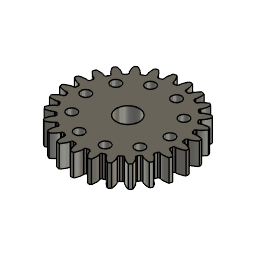
Main gear (Autodesk Fusion 360 design; units mm, degrees)
part number: 2026-05-08-17-31-43-682
Autodesk Fusion 360 part; units mm, degrees
(part 1 of 7)
sketch "Base Circle" plane through (0, 0, 0) normal (0, 0, 1) x (1, 0, 0)
  circle A0 centre (0, 0) radius 11.343
  circle A1 centre (0, 0) radius 2.6
extrude "Extrude6" add sketch "Base Circle" along normal blind 5
sketch "Gear Tooth" plane through (0, 0, 0) normal (0, 0, 1) x (1, 0, 0)
  spline S0 degree 5 poles (11.7116, -0.9005) (11.7167, -0.9009) (11.7269, -0.9015) (11.7422, -0.9021) (11.7626, -0.9022) (11.7882, -0.9014) (11.8137, -0.8998) (11.8394, -0.8977) (11.865, -0.8955) (11.8906, -0.893) (11.9163, -0.8904) (11.9419, -0.8876) (11.9676, -0.8845) (11.9933, -0.8811) (12.0189, -0.8773) (12.0446, -0.8732) (12.0703, -0.8688) (12.096, -0.8641) (12.1216, -0.8593) (12.1473, -0.8543) (12.173, -0.8491) (12.1987, -0.8437) (12.2244, -0.838) (12.25, -0.8322) (12.2757, -0.8262) (12.3014, -0.8199) (12.3271, -0.8135) (12.3527, -0.8068) (12.3784, -0.8) (12.404, -0.793) (12.4297, -0.7859) (12.4553, -0.7785) (12.4809, -0.771) (12.5066, -0.7633) (12.5322, -0.7555) (12.5578, -0.7475) (12.5834, -0.7393) (12.609, -0.7309) (12.6345, -0.7224) (12.6601, -0.7137) (12.6857, -0.7049) (12.7112, -0.6959) (12.7367, -0.6868) (12.7623, -0.6775) (12.7878, -0.668) (12.8133, -0.6584) (12.8387, -0.6487) (12.8642, -0.6388) (12.8897, -0.6287) (12.9151, -0.6185) (12.9405, -0.6082) (12.9659, -0.5977) (12.9913, -0.5871) (13.0167, -0.5764) (13.0421, -0.5655) (13.0674, -0.5544) (13.0928, -0.5433) (13.1181, -0.532) (13.1434, -0.5205) (13.1687, -0.5089) (13.1939, -0.4972) (13.2192, -0.4854) (13.2444, -0.4734) (13.2696, -0.4613) (13.2948, -0.449) (13.32, -0.4366) (13.3451, -0.4241) (13.3702, -0.4115) (13.3953, -0.3987) (13.4204, -0.3858) (13.4455, -0.3728) (13.4655, -0.3623) (13.4805, -0.3544) (13.4906, -0.349) (13.4956, -0.3464) knots 0 0 0 0 0 0 0.01428571 0.02857143 0.04285714 0.05714286 0.07142857 0.08571429 0.1 0.11428571 0.12857143 0.14285714 0.15714286 0.17142857 0.18571429 0.2 0.21428571 0.22857143 0.24285714 0.25714286 0.27142857 0.28571429 0.3 0.31428571 0.32857143 0.34285714 0.35714286 0.37142857 0.38571429 0.4 0.41428571 0.42857143 0.44285714 0.45714286 0.47142857 0.48571429 0.5 0.51428571 0.52857143 0.54285714 0.55714286 0.57142857 0.58571429 0.6 0.61428571 0.62857143 0.64285714 0.65714286 0.67142857 0.68571429 0.7 0.71428571 0.72857143 0.74285714 0.75714286 0.77142857 0.78571429 0.8 0.81428571 0.82857143 0.84285714 0.85714286 0.87142857 0.88571429 0.9 0.91428571 0.92857143 0.94285714 0.95714286 0.97142857 0.98571429 1 1 1 1 1 1
  spline S1 degree 5 poles (11.7116, 0.9005) (11.7167, 0.9009) (11.7269, 0.9015) (11.7422, 0.9021) (11.7626, 0.9022) (11.7882, 0.9014) (11.8137, 0.8998) (11.8394, 0.8977) (11.865, 0.8955) (11.8906, 0.893) (11.9163, 0.8904) (11.9419, 0.8876) (11.9676, 0.8845) (11.9933, 0.8811) (12.0189, 0.8773) (12.0446, 0.8732) (12.0703, 0.8688) (12.096, 0.8641) (12.1216, 0.8593) (12.1473, 0.8543) (12.173, 0.8491) (12.1987, 0.8437) (12.2244, 0.838) (12.25, 0.8322) (12.2757, 0.8262) (12.3014, 0.8199) (12.3271, 0.8135) (12.3527, 0.8068) (12.3784, 0.8) (12.404, 0.793) (12.4297, 0.7859) (12.4553, 0.7785) (12.4809, 0.771) (12.5066, 0.7633) (12.5322, 0.7555) (12.5578, 0.7475) (12.5834, 0.7393) (12.609, 0.7309) (12.6345, 0.7224) (12.6601, 0.7137) (12.6857, 0.7049) (12.7112, 0.6959) (12.7367, 0.6868) (12.7623, 0.6775) (12.7878, 0.668) (12.8133, 0.6584) (12.8387, 0.6487) (12.8642, 0.6388) (12.8897, 0.6287) (12.9151, 0.6185) (12.9405, 0.6082) (12.9659, 0.5977) (12.9913, 0.5871) (13.0167, 0.5764) (13.0421, 0.5655) (13.0674, 0.5544) (13.0928, 0.5433) (13.1181, 0.532) (13.1434, 0.5205) (13.1687, 0.5089) (13.1939, 0.4972) (13.2192, 0.4854) (13.2444, 0.4734) (13.2696, 0.4613) (13.2948, 0.449) (13.32, 0.4366) (13.3451, 0.4241) (13.3702, 0.4115) (13.3953, 0.3987) (13.4204, 0.3858) (13.4455, 0.3728) (13.4655, 0.3623) (13.4805, 0.3544) (13.4906, 0.349) (13.4956, 0.3464) knots 0 0 0 0 0 0 0.01428571 0.02857143 0.04285714 0.05714286 0.07142857 0.08571429 0.1 0.11428571 0.12857143 0.14285714 0.15714286 0.17142857 0.18571429 0.2 0.21428571 0.22857143 0.24285714 0.25714286 0.27142857 0.28571429 0.3 0.31428571 0.32857143 0.34285714 0.35714286 0.37142857 0.38571429 0.4 0.41428571 0.42857143 0.44285714 0.45714286 0.47142857 0.48571429 0.5 0.51428571 0.52857143 0.54285714 0.55714286 0.57142857 0.58571429 0.6 0.61428571 0.62857143 0.64285714 0.65714286 0.67142857 0.68571429 0.7 0.71428571 0.72857143 0.74285714 0.75714286 0.77142857 0.78571429 0.8 0.81428571 0.82857143 0.84285714 0.85714286 0.87142857 0.88571429 0.9 0.91428571 0.92857143 0.94285714 0.95714286 0.97142857 0.98571429 1 1 1 1 1 1
  arc A0 (13.4956, -0.3464) -> (13.4956, 0.3464) centre (0, 0) ccw
  line L0 (11.2996, -0.8688) -> (11.7116, -0.9005)
  line L1 (11.2996, 0.8688) -> (11.7116, 0.9005)
  line L2 (11.2996, -0.8688) -> (11.2996, 0.8688)
  point P0 (11.8374, -0.8978)
  point P1 (11.964, -0.8849)
  point P2 (12.0911, -0.865)
  point P3 (12.2185, -0.8393)
  point P4 (12.3461, -0.8085)
  point P5 (12.4739, -0.7731)
  point P6 (12.6018, -0.7332)
  point P7 (12.7297, -0.6892)
  point P8 (12.8576, -0.6413)
  point P9 (12.9855, -0.5895)
  point P10 (13.1133, -0.5341)
  point P11 (13.2409, -0.475)
  point P12 (13.3684, -0.4124)
  point P13 (11.8374, 0.8978)
  point P14 (11.964, 0.8849)
  point P15 (12.0911, 0.865)
  point P16 (12.2185, 0.8393)
  point P17 (12.3461, 0.8085)
  point P18 (12.4739, 0.7731)
  point P19 (12.6018, 0.7332)
  point P20 (12.7297, 0.6892)
  point P21 (12.8576, 0.6413)
  point P22 (12.9855, 0.5895)
  point P23 (13.1133, 0.5341)
  point P24 (13.2409, 0.475)
  point P25 (13.3684, 0.4124)
extrude "Extrude7" add sketch "Gear Tooth" along normal blind 5
fillet "Fillet3" radius 0.3 2 edges at (11.3096, -0.8696, 2.5) (11.3096, 0.8696, 2.5)
pattern_circular "C-Pattern3" count 25 over 360 about axis through (0, 0, 0) along (0, 0, 1) of "Extrude7", "Fillet3"
sketch "Diametrial Pitch Circle" plane through (0, 0, 0) normal (0, 0, 1) x (1, 0, 0)
  circle A0 centre (0, 0) radius 12.5 construction
sketch "gauri flaps" plane through (0, 0, 5) normal (0, 0, 1) x (-1, 0, 0)
  arc A0 (-11.2176, 1.6819) -> (-11.2835, 1.1607) centre (0, 0) ccw
  arc A1 (-11.6049, 0.8923) -> (-11.2835, 1.1607) centre (-11.5819, 1.1914) ccw
  line L0 (-11.6049, 0.8923) -> (-11.7116, 0.9005)
  spline S0 degree 5 poles (-11.7116, 0.9005) (-11.7167, 0.9009) (-11.7269, 0.9015) (-11.7422, 0.9021) (-11.7626, 0.9022) (-11.7882, 0.9014) (-11.8137, 0.8998) (-11.8394, 0.8977) (-11.865, 0.8955) (-11.8906, 0.893) (-11.9163, 0.8904) (-11.9419, 0.8876) (-11.9676, 0.8845) (-11.9933, 0.8811) (-12.0189, 0.8773) (-12.0446, 0.8732) (-12.0703, 0.8688) (-12.096, 0.8641) (-12.1216, 0.8593) (-12.1473, 0.8543) (-12.173, 0.8491) (-12.1987, 0.8437) (-12.2244, 0.838) (-12.25, 0.8322) (-12.2757, 0.8262) (-12.3014, 0.8199) (-12.3271, 0.8135) (-12.3527, 0.8068) (-12.3784, 0.8) (-12.404, 0.793) (-12.4297, 0.7859) (-12.4553, 0.7785) (-12.4809, 0.771) (-12.5066, 0.7633) (-12.5322, 0.7555) (-12.5578, 0.7475) (-12.5834, 0.7393) (-12.609, 0.7309) (-12.6345, 0.7224) (-12.6601, 0.7137) (-12.6857, 0.7049) (-12.7112, 0.6959) (-12.7367, 0.6868) (-12.7623, 0.6775) (-12.7878, 0.668) (-12.8133, 0.6584) (-12.8387, 0.6487) (-12.8642, 0.6388) (-12.8897, 0.6287) (-12.9151, 0.6185) (-12.9405, 0.6082) (-12.9659, 0.5977) (-12.9913, 0.5871) (-13.0167, 0.5764) (-13.0421, 0.5655) (-13.0674, 0.5544) (-13.0928, 0.5433) (-13.1181, 0.532) (-13.1434, 0.5205) (-13.1687, 0.5089) (-13.1939, 0.4972) (-13.2192, 0.4854) (-13.2444, 0.4734) (-13.2696, 0.4613) (-13.2948, 0.449) (-13.32, 0.4366) (-13.3451, 0.4241) (-13.3702, 0.4115) (-13.3953, 0.3987) (-13.4204, 0.3858) (-13.4455, 0.3728) (-13.4655, 0.3623) (-13.4805, 0.3544) (-13.4906, 0.349) (-13.4956, 0.3464) knots 0 0 0 0 0 0 0.01428571 0.02857143 0.04285714 0.05714286 0.07142857 0.08571429 0.1 0.11428571 0.12857143 0.14285714 0.15714286 0.17142857 0.18571429 0.2 0.21428571 0.22857143 0.24285714 0.25714286 0.27142857 0.28571429 0.3 0.31428571 0.32857143 0.34285714 0.35714286 0.37142857 0.38571429 0.4 0.41428571 0.42857143 0.44285714 0.45714286 0.47142857 0.48571429 0.5 0.51428571 0.52857143 0.54285714 0.55714286 0.57142857 0.58571429 0.6 0.61428571 0.62857143 0.64285714 0.65714286 0.67142857 0.68571429 0.7 0.71428571 0.72857143 0.74285714 0.75714286 0.77142857 0.78571429 0.8 0.81428571 0.82857143 0.84285714 0.85714286 0.87142857 0.88571429 0.9 0.91428571 0.92857143 0.94285714 0.95714286 0.97142857 0.98571429 1 1 1 1 1 1
  arc A2 (-13.4956, 0.3464) -> (-13.4956, -0.3464) centre (0, 0) ccw
  spline S1 degree 5 poles (-13.4956, -0.3464) (-13.4906, -0.349) (-13.4805, -0.3544) (-13.4655, -0.3623) (-13.4455, -0.3728) (-13.4204, -0.3858) (-13.3953, -0.3987) (-13.3702, -0.4115) (-13.3451, -0.4241) (-13.32, -0.4366) (-13.2948, -0.449) (-13.2696, -0.4613) (-13.2444, -0.4734) (-13.2192, -0.4854) (-13.1939, -0.4972) (-13.1687, -0.5089) (-13.1434, -0.5205) (-13.1181, -0.532) (-13.0928, -0.5433) (-13.0674, -0.5544) (-13.0421, -0.5655) (-13.0167, -0.5764) (-12.9913, -0.5871) (-12.9659, -0.5977) (-12.9405, -0.6082) (-12.9151, -0.6185) (-12.8897, -0.6287) (-12.8642, -0.6388) (-12.8387, -0.6487) (-12.8133, -0.6584) (-12.7878, -0.668) (-12.7623, -0.6775) (-12.7367, -0.6868) (-12.7112, -0.6959) (-12.6857, -0.7049) (-12.6601, -0.7137) (-12.6345, -0.7224) (-12.609, -0.7309) (-12.5834, -0.7393) (-12.5578, -0.7475) (-12.5322, -0.7555) (-12.5066, -0.7633) (-12.4809, -0.771) (-12.4553, -0.7785) (-12.4297, -0.7859) (-12.404, -0.793) (-12.3784, -0.8) (-12.3527, -0.8068) (-12.3271, -0.8135) (-12.3014, -0.8199) (-12.2757, -0.8262) (-12.25, -0.8322) (-12.2244, -0.838) (-12.1987, -0.8437) (-12.173, -0.8491) (-12.1473, -0.8543) (-12.1216, -0.8593) (-12.096, -0.8641) (-12.0703, -0.8688) (-12.0446, -0.8732) (-12.0189, -0.8773) (-11.9933, -0.8811) (-11.9676, -0.8845) (-11.9419, -0.8876) (-11.9163, -0.8904) (-11.8906, -0.893) (-11.865, -0.8955) (-11.8394, -0.8977) (-11.8137, -0.8998) (-11.7882, -0.9014) (-11.7626, -0.9022) (-11.7422, -0.9021) (-11.7269, -0.9015) (-11.7167, -0.9009) (-11.7116, -0.9005) knots -1 -1 -1 -1 -1 -1 -0.98571429 -0.97142857 -0.95714286 -0.94285714 -0.92857143 -0.91428571 -0.9 -0.88571429 -0.87142857 -0.85714286 -0.84285714 -0.82857143 -0.81428571 -0.8 -0.78571429 -0.77142857 -0.75714286 -0.74285714 -0.72857143 -0.71428571 -0.7 -0.68571429 -0.67142857 -0.65714286 -0.64285714 -0.62857143 -0.61428571 -0.6 -0.58571429 -0.57142857 -0.55714286 -0.54285714 -0.52857143 -0.51428571 -0.5 -0.48571429 -0.47142857 -0.45714286 -0.44285714 -0.42857143 -0.41428571 -0.4 -0.38571429 -0.37142857 -0.35714286 -0.34285714 -0.32857143 -0.31428571 -0.3 -0.28571429 -0.27142857 -0.25714286 -0.24285714 -0.22857143 -0.21428571 -0.2 -0.18571429 -0.17142857 -0.15714286 -0.14285714 -0.12857143 -0.11428571 -0.1 -0.08571429 -0.07142857 -0.05714286 -0.04285714 -0.02857143 -0.01428571 0 0 0 0 0 0
  line L1 (-11.7116, -0.9005) -> (-11.6049, -0.8923)
  arc A3 (-11.2835, -1.1607) -> (-11.6049, -0.8923) centre (-11.5819, -1.1914) ccw
  arc A4 (-11.2835, -1.1607) -> (-11.2176, -1.6819) centre (0, 0) ccw
  arc A5 (-11.4622, -2.0218) -> (-11.2176, -1.6819) centre (-11.5143, -1.7263) ccw
  line L2 (-11.4622, -2.0218) -> (-11.5676, -2.0404)
  spline S2 degree 5 poles (-11.5676, -2.0404) (-11.5726, -2.0413) (-11.5827, -2.0432) (-11.5976, -2.0464) (-11.6174, -2.0514) (-11.642, -2.0586) (-11.6664, -2.0665) (-11.6907, -2.0748) (-11.7149, -2.0834) (-11.7391, -2.0921) (-11.7633, -2.101) (-11.7875, -2.1101) (-11.8116, -2.1195) (-11.8356, -2.1292) (-11.8595, -2.1393) (-11.8833, -2.1496) (-11.9071, -2.1603) (-11.9308, -2.1712) (-11.9545, -2.1822) (-11.9781, -2.1935) (-12.0017, -2.2049) (-12.0253, -2.2165) (-12.0487, -2.2284) (-12.0722, -2.2404) (-12.0955, -2.2526) (-12.1188, -2.2651) (-12.1421, -2.2777) (-12.1653, -2.2905) (-12.1884, -2.3035) (-12.2115, -2.3166) (-12.2346, -2.33) (-12.2576, -2.3434) (-12.2806, -2.3571) (-12.3035, -2.3709) (-12.3263, -2.3849) (-12.3491, -2.399) (-12.3719, -2.4133) (-12.3946, -2.4278) (-12.4172, -2.4424) (-12.4399, -2.4571) (-12.4624, -2.4721) (-12.4849, -2.4871) (-12.5074, -2.5023) (-12.5298, -2.5177) (-12.5521, -2.5332) (-12.5744, -2.5488) (-12.5967, -2.5646) (-12.6189, -2.5805) (-12.6411, -2.5965) (-12.6632, -2.6127) (-12.6852, -2.6291) (-12.7072, -2.6455) (-12.7292, -2.6621) (-12.7511, -2.6789) (-12.773, -2.6957) (-12.7948, -2.7127) (-12.8165, -2.7298) (-12.8382, -2.7471) (-12.8599, -2.7645) (-12.8815, -2.782) (-12.9031, -2.7996) (-12.9246, -2.8174) (-12.946, -2.8352) (-12.9674, -2.8532) (-12.9888, -2.8714) (-13.0101, -2.8896) (-13.0313, -2.908) (-13.0525, -2.9265) (-13.0737, -2.9451) (-13.0948, -2.9638) (-13.1158, -2.9827) (-13.1326, -2.9978) (-13.1452, -3.0092) (-13.1535, -3.0169) (-13.1577, -3.0207) knots 0 0 0 0 0 0 0.01428571 0.02857143 0.04285714 0.05714286 0.07142857 0.08571429 0.1 0.11428571 0.12857143 0.14285714 0.15714286 0.17142857 0.18571429 0.2 0.21428571 0.22857143 0.24285714 0.25714286 0.27142857 0.28571429 0.3 0.31428571 0.32857143 0.34285714 0.35714286 0.37142857 0.38571429 0.4 0.41428571 0.42857143 0.44285714 0.45714286 0.47142857 0.48571429 0.5 0.51428571 0.52857143 0.54285714 0.55714286 0.57142857 0.58571429 0.6 0.61428571 0.62857143 0.64285714 0.65714286 0.67142857 0.68571429 0.7 0.71428571 0.72857143 0.74285714 0.75714286 0.77142857 0.78571429 0.8 0.81428571 0.82857143 0.84285714 0.85714286 0.87142857 0.88571429 0.9 0.91428571 0.92857143 0.94285714 0.95714286 0.97142857 0.98571429 1 1 1 1 1 1
  arc A6 (-13.1577, -3.0207) -> (-12.9854, -3.6917) centre (0, 0) ccw
  spline S3 degree 5 poles (-12.9854, -3.6917) (-12.9799, -3.693) (-12.9689, -3.6957) (-12.9524, -3.6997) (-12.9304, -3.7049) (-12.9028, -3.7112) (-12.8753, -3.7175) (-12.8478, -3.7236) (-12.8204, -3.7296) (-12.7929, -3.7355) (-12.7654, -3.7412) (-12.738, -3.7468) (-12.7106, -3.7522) (-12.6832, -3.7576) (-12.6558, -3.7628) (-12.6284, -3.7678) (-12.601, -3.7728) (-12.5737, -3.7776) (-12.5463, -3.7822) (-12.519, -3.7868) (-12.4917, -3.7911) (-12.4644, -3.7954) (-12.4372, -3.7995) (-12.4099, -3.8035) (-12.3827, -3.8073) (-12.3555, -3.811) (-12.3283, -3.8145) (-12.3012, -3.8179) (-12.2741, -3.8212) (-12.247, -3.8243) (-12.2199, -3.8272) (-12.1928, -3.83) (-12.1658, -3.8327) (-12.1388, -3.8352) (-12.1118, -3.8375) (-12.0849, -3.8397) (-12.0579, -3.8418) (-12.0311, -3.8437) (-12.0042, -3.8454) (-11.9774, -3.847) (-11.9506, -3.8484) (-11.9238, -3.8496) (-11.8971, -3.8507) (-11.8704, -3.8516) (-11.8437, -3.8523) (-11.8171, -3.8529) (-11.7905, -3.8533) (-11.764, -3.8535) (-11.7375, -3.8535) (-11.711, -3.8534) (-11.6846, -3.8531) (-11.6582, -3.8525) (-11.6319, -3.8518) (-11.6056, -3.8508) (-11.5794, -3.8497) (-11.5532, -3.8484) (-11.5271, -3.8468) (-11.501, -3.8451) (-11.475, -3.8432) (-11.4491, -3.8411) (-11.4232, -3.8387) (-11.3974, -3.836) (-11.3716, -3.8329) (-11.346, -3.8296) (-11.3205, -3.8259) (-11.295, -3.8221) (-11.2695, -3.818) (-11.2441, -3.8139) (-11.2188, -3.8095) (-11.1937, -3.8046) (-11.1687, -3.7991) (-11.1489, -3.794) (-11.1343, -3.7896) (-11.1245, -3.7864) (-11.1197, -3.7847) knots -1 -1 -1 -1 -1 -1 -0.98571429 -0.97142857 -0.95714286 -0.94285714 -0.92857143 -0.91428571 -0.9 -0.88571429 -0.87142857 -0.85714286 -0.84285714 -0.82857143 -0.81428571 -0.8 -0.78571429 -0.77142857 -0.75714286 -0.74285714 -0.72857143 -0.71428571 -0.7 -0.68571429 -0.67142857 -0.65714286 -0.64285714 -0.62857143 -0.61428571 -0.6 -0.58571429 -0.57142857 -0.55714286 -0.54285714 -0.52857143 -0.51428571 -0.5 -0.48571429 -0.47142857 -0.45714286 -0.44285714 -0.42857143 -0.41428571 -0.4 -0.38571429 -0.37142857 -0.35714286 -0.34285714 -0.32857143 -0.31428571 -0.3 -0.28571429 -0.27142857 -0.25714286 -0.24285714 -0.22857143 -0.21428571 -0.2 -0.18571429 -0.17142857 -0.15714286 -0.14285714 -0.12857143 -0.11428571 -0.1 -0.08571429 -0.07142857 -0.05714286 -0.04285714 -0.02857143 -0.01428571 0 0 0 0 0 0
  line L3 (-11.1197, -3.7847) -> (-11.0184, -3.7503)
  arc A7 (-10.6403, -3.9303) -> (-11.0184, -3.7503) centre (-10.9217, -4.0343) ccw
  arc A8 (-10.6403, -3.9303) -> (-10.4469, -4.4187) centre (0, 0) ccw
  arc A9 (-10.5993, -4.8088) -> (-10.4469, -4.4187) centre (-10.7232, -4.5356) ccw
  line L4 (-10.5993, -4.8088) -> (-10.6968, -4.853)
  spline S4 degree 5 poles (-10.6968, -4.853) (-10.7014, -4.8551) (-10.7107, -4.8595) (-10.7244, -4.8663) (-10.7423, -4.8761) (-10.7643, -4.8891) (-10.7859, -4.9028) (-10.8074, -4.917) (-10.8288, -4.9313) (-10.85, -4.9458) (-10.8713, -4.9604) (-10.8924, -4.9752) (-10.9134, -4.9903) (-10.9342, -5.0057) (-10.9549, -5.0214) (-10.9754, -5.0374) (-10.9958, -5.0536) (-11.0161, -5.07) (-11.0362, -5.0866) (-11.0563, -5.1034) (-11.0763, -5.1203) (-11.0962, -5.1375) (-11.116, -5.1547) (-11.1357, -5.1722) (-11.1553, -5.1899) (-11.1748, -5.2077) (-11.1942, -5.2258) (-11.2135, -5.2439) (-11.2327, -5.2623) (-11.2518, -5.2807) (-11.2708, -5.2994) (-11.2897, -5.3182) (-11.3086, -5.3371) (-11.3273, -5.3562) (-11.346, -5.3754) (-11.3646, -5.3948) (-11.383, -5.4143) (-11.4014, -5.4339) (-11.4197, -5.4537) (-11.438, -5.4736) (-11.4561, -5.4937) (-11.4742, -5.5138) (-11.4921, -5.5342) (-11.51, -5.5546) (-11.5278, -5.5752) (-11.5455, -5.5959) (-11.5632, -5.6167) (-11.5807, -5.6376) (-11.5982, -5.6587) (-11.6156, -5.6799) (-11.6329, -5.7012) (-11.6501, -5.7226) (-11.6672, -5.7441) (-11.6843, -5.7658) (-11.7013, -5.7875) (-11.7182, -5.8094) (-11.735, -5.8314) (-11.7517, -5.8535) (-11.7684, -5.8757) (-11.785, -5.8981) (-11.8015, -5.9205) (-11.8179, -5.9431) (-11.8342, -5.9657) (-11.8505, -5.9885) (-11.8666, -6.0113) (-11.8827, -6.0343) (-11.8987, -6.0574) (-11.9147, -6.0806) (-11.9305, -6.1038) (-11.9463, -6.1272) (-11.962, -6.1507) (-11.9745, -6.1696) (-11.9838, -6.1838) (-11.99, -6.1933) (-11.9931, -6.198) knots 0 0 0 0 0 0 0.01428571 0.02857143 0.04285714 0.05714286 0.07142857 0.08571429 0.1 0.11428571 0.12857143 0.14285714 0.15714286 0.17142857 0.18571429 0.2 0.21428571 0.22857143 0.24285714 0.25714286 0.27142857 0.28571429 0.3 0.31428571 0.32857143 0.34285714 0.35714286 0.37142857 0.38571429 0.4 0.41428571 0.42857143 0.44285714 0.45714286 0.47142857 0.48571429 0.5 0.51428571 0.52857143 0.54285714 0.55714286 0.57142857 0.58571429 0.6 0.61428571 0.62857143 0.64285714 0.65714286 0.67142857 0.68571429 0.7 0.71428571 0.72857143 0.74285714 0.75714286 0.77142857 0.78571429 0.8 0.81428571 0.82857143 0.84285714 0.85714286 0.87142857 0.88571429 0.9 0.91428571 0.92857143 0.94285714 0.95714286 0.97142857 0.98571429 1 1 1 1 1 1
  arc A10 (-11.9931, -6.198) -> (-11.6594, -6.8051) centre (0, 0) ccw
  spline S5 degree 5 poles (-11.6594, -6.8051) (-11.6537, -6.805) (-11.6424, -6.8048) (-11.6254, -6.8046) (-11.6028, -6.8041) (-11.5745, -6.8035) (-11.5463, -6.8027) (-11.5182, -6.8018) (-11.4901, -6.8007) (-11.462, -6.7996) (-11.434, -6.7983) (-11.406, -6.7969) (-11.3781, -6.7954) (-11.3502, -6.7937) (-11.3224, -6.7919) (-11.2946, -6.79) (-11.2669, -6.788) (-11.2392, -6.7858) (-11.2116, -6.7836) (-11.184, -6.7811) (-11.1564, -6.7786) (-11.129, -6.7759) (-11.1015, -6.7731) (-11.0742, -6.7702) (-11.0469, -6.7671) (-11.0196, -6.7639) (-10.9924, -6.7606) (-10.9653, -6.7571) (-10.9382, -6.7535) (-10.9111, -6.7498) (-10.8842, -6.7459) (-10.8573, -6.7419) (-10.8304, -6.7378) (-10.8037, -6.7335) (-10.7769, -6.7291) (-10.7503, -6.7245) (-10.7237, -6.7198) (-10.6972, -6.7149) (-10.6707, -6.7099) (-10.6444, -6.7048) (-10.6181, -6.6995) (-10.5918, -6.694) (-10.5657, -6.6884) (-10.5396, -6.6826) (-10.5136, -6.6767) (-10.4877, -6.6706) (-10.4618, -6.6644) (-10.4361, -6.658) (-10.4104, -6.6515) (-10.3848, -6.6447) (-10.3593, -6.6379) (-10.3339, -6.6308) (-10.3086, -6.6235) (-10.2834, -6.6161) (-10.2582, -6.6084) (-10.2332, -6.6006) (-10.2083, -6.5927) (-10.1835, -6.5845) (-10.1587, -6.5762) (-10.1341, -6.5677) (-10.1096, -6.5589) (-10.0853, -6.5499) (-10.0612, -6.5405) (-10.0372, -6.5309) (-10.0133, -6.521) (-9.9896, -6.5109) (-9.966, -6.5007) (-9.9424, -6.4904) (-9.919, -6.4798) (-9.8958, -6.4689) (-9.873, -6.4573) (-9.8551, -6.4474) (-9.842, -6.4395) (-9.8334, -6.434) (-9.8291, -6.4312) knots -1 -1 -1 -1 -1 -1 -0.98571429 -0.97142857 -0.95714286 -0.94285714 -0.92857143 -0.91428571 -0.9 -0.88571429 -0.87142857 -0.85714286 -0.84285714 -0.82857143 -0.81428571 -0.8 -0.78571429 -0.77142857 -0.75714286 -0.74285714 -0.72857143 -0.71428571 -0.7 -0.68571429 -0.67142857 -0.65714286 -0.64285714 -0.62857143 -0.61428571 -0.6 -0.58571429 -0.57142857 -0.55714286 -0.54285714 -0.52857143 -0.51428571 -0.5 -0.48571429 -0.47142857 -0.45714286 -0.44285714 -0.42857143 -0.41428571 -0.4 -0.38571429 -0.37142857 -0.35714286 -0.34285714 -0.32857143 -0.31428571 -0.3 -0.28571429 -0.27142857 -0.25714286 -0.24285714 -0.22857143 -0.21428571 -0.2 -0.18571429 -0.17142857 -0.15714286 -0.14285714 -0.12857143 -0.11428571 -0.1 -0.08571429 -0.07142857 -0.05714286 -0.04285714 -0.02857143 -0.01428571 0 0 0 0 0 0
  line L5 (-9.8291, -6.4312) -> (-9.7396, -6.3726)
  arc A11 (-9.3286, -6.453) -> (-9.7396, -6.3726) centre (-9.5753, -6.6236) ccw
  arc A12 (-9.3286, -6.453) -> (-9.0198, -6.878) centre (0, 0) ccw
  arc A13 (-9.0704, -7.2937) -> (-9.0198, -6.878) centre (-9.2584, -7.0599) ccw
  line L6 (-9.0704, -7.2937) -> (-9.1538, -7.3607)
  spline S6 degree 5 poles (-9.1538, -7.3607) (-9.1578, -7.3639) (-9.1657, -7.3704) (-9.1772, -7.3805) (-9.1922, -7.3944) (-9.2102, -7.4125) (-9.2278, -7.4312) (-9.2451, -7.4502) (-9.2622, -7.4694) (-9.2792, -7.4887) (-9.2961, -7.5081) (-9.3129, -7.5278) (-9.3295, -7.5476) (-9.3458, -7.5677) (-9.362, -7.588) (-9.3779, -7.6086) (-9.3936, -7.6294) (-9.4091, -7.6503) (-9.4245, -7.6714) (-9.4398, -7.6927) (-9.455, -7.7141) (-9.47, -7.7356) (-9.4849, -7.7572) (-9.4996, -7.7791) (-9.5142, -7.8011) (-9.5286, -7.8232) (-9.5429, -7.8455) (-9.5571, -7.8679) (-9.5711, -7.8904) (-9.585, -7.913) (-9.5988, -7.9358) (-9.6125, -7.9587) (-9.626, -7.9817) (-9.6394, -8.0049) (-9.6527, -8.0281) (-9.6659, -8.0515) (-9.6789, -8.075) (-9.6919, -8.0986) (-9.7047, -8.1223) (-9.7174, -8.1462) (-9.73, -8.1701) (-9.7424, -8.1941) (-9.7548, -8.2183) (-9.767, -8.2425) (-9.7792, -8.2669) (-9.7912, -8.2913) (-9.8031, -8.3159) (-9.8149, -8.3405) (-9.8266, -8.3653) (-9.8381, -8.3901) (-9.8496, -8.415) (-9.8609, -8.4401) (-9.8722, -8.4652) (-9.8833, -8.4904) (-9.8944, -8.5157) (-9.9053, -8.5411) (-9.9161, -8.5666) (-9.9268, -8.5922) (-9.9374, -8.6178) (-9.9479, -8.6436) (-9.9583, -8.6694) (-9.9686, -8.6953) (-9.9788, -8.7213) (-9.9889, -8.7474) (-9.9989, -8.7736) (-10.0087, -8.7998) (-10.0185, -8.8262) (-10.0282, -8.8526) (-10.0377, -8.8791) (-10.0472, -8.9057) (-10.0566, -8.9323) (-10.064, -8.9537) (-10.0695, -8.9698) (-10.0731, -8.9805) (-10.0749, -8.9858) knots 0 0 0 0 0 0 0.01428571 0.02857143 0.04285714 0.05714286 0.07142857 0.08571429 0.1 0.11428571 0.12857143 0.14285714 0.15714286 0.17142857 0.18571429 0.2 0.21428571 0.22857143 0.24285714 0.25714286 0.27142857 0.28571429 0.3 0.31428571 0.32857143 0.34285714 0.35714286 0.37142857 0.38571429 0.4 0.41428571 0.42857143 0.44285714 0.45714286 0.47142857 0.48571429 0.5 0.51428571 0.52857143 0.54285714 0.55714286 0.57142857 0.58571429 0.6 0.61428571 0.62857143 0.64285714 0.65714286 0.67142857 0.68571429 0.7 0.71428571 0.72857143 0.74285714 0.75714286 0.77142857 0.78571429 0.8 0.81428571 0.82857143 0.84285714 0.85714286 0.87142857 0.88571429 0.9 0.91428571 0.92857143 0.94285714 0.95714286 0.97142857 0.98571429 1 1 1 1 1 1
  arc A14 (-10.0749, -8.9858) -> (-9.6007, -9.4908) centre (0, 0) ccw
  spline S7 degree 5 poles (-9.6007, -9.4908) (-9.5953, -9.4894) (-9.5843, -9.4864) (-9.5679, -9.4819) (-9.5461, -9.4758) (-9.5189, -9.4682) (-9.4918, -9.4604) (-9.4648, -9.4525) (-9.4378, -9.4445) (-9.4109, -9.4364) (-9.3841, -9.4282) (-9.3574, -9.4199) (-9.3307, -9.4115) (-9.3041, -9.403) (-9.2776, -9.3943) (-9.2512, -9.3856) (-9.2248, -9.3767) (-9.1985, -9.3677) (-9.1723, -9.3586) (-9.1462, -9.3494) (-9.1202, -9.3401) (-9.0942, -9.3307) (-9.0684, -9.3212) (-9.0426, -9.3115) (-9.0169, -9.3018) (-8.9913, -9.2919) (-8.9658, -9.2819) (-8.9403, -9.2718) (-8.915, -9.2616) (-8.8897, -9.2512) (-8.8646, -9.2408) (-8.8395, -9.2302) (-8.8146, -9.2195) (-8.7897, -9.2087) (-8.7649, -9.1978) (-8.7402, -9.1867) (-8.7157, -9.1755) (-8.6912, -9.1642) (-8.6668, -9.1528) (-8.6426, -9.1413) (-8.6184, -9.1296) (-8.5943, -9.1178) (-8.5704, -9.1058) (-8.5466, -9.0938) (-8.5229, -9.0816) (-8.4993, -9.0692) (-8.4758, -9.0568) (-8.4524, -9.0442) (-8.4292, -9.0314) (-8.4061, -9.0186) (-8.3831, -9.0056) (-8.3602, -8.9924) (-8.3375, -8.9791) (-8.3149, -8.9656) (-8.2925, -8.9519) (-8.2702, -8.9382) (-8.2481, -8.9242) (-8.226, -8.9102) (-8.2042, -8.896) (-8.1824, -8.8816) (-8.1609, -8.867) (-8.1396, -8.8522) (-8.1185, -8.8372) (-8.0977, -8.8219) (-8.077, -8.8063) (-8.0566, -8.7907) (-8.0362, -8.7749) (-8.016, -8.759) (-7.9959, -8.743) (-7.9762, -8.7266) (-7.957, -8.7098) (-7.9421, -8.6957) (-7.9314, -8.6848) (-7.9244, -8.6773) (-7.921, -8.6736) knots -1 -1 -1 -1 -1 -1 -0.98571429 -0.97142857 -0.95714286 -0.94285714 -0.92857143 -0.91428571 -0.9 -0.88571429 -0.87142857 -0.85714286 -0.84285714 -0.82857143 -0.81428571 -0.8 -0.78571429 -0.77142857 -0.75714286 -0.74285714 -0.72857143 -0.71428571 -0.7 -0.68571429 -0.67142857 -0.65714286 -0.64285714 -0.62857143 -0.61428571 -0.6 -0.58571429 -0.57142857 -0.55714286 -0.54285714 -0.52857143 -0.51428571 -0.5 -0.48571429 -0.47142857 -0.45714286 -0.44285714 -0.42857143 -0.41428571 -0.4 -0.38571429 -0.37142857 -0.35714286 -0.34285714 -0.32857143 -0.31428571 -0.3 -0.28571429 -0.27142857 -0.25714286 -0.24285714 -0.22857143 -0.21428571 -0.2 -0.18571429 -0.17142857 -0.15714286 -0.14285714 -0.12857143 -0.11428571 -0.1 -0.08571429 -0.07142857 -0.05714286 -0.04285714 -0.02857143 -0.01428571 0 0 0 0 0 0
  line L7 (-7.921, -8.6736) -> (-7.8488, -8.5945)
  arc A15 (-7.4307, -8.5702) -> (-7.8488, -8.5945) centre (-7.6273, -8.7968) ccw
  arc A16 (-7.4307, -8.5702) -> (-7.026, -8.905) centre (0, 0) ccw
  arc A17 (-6.9716, -9.3202) -> (-7.026, -8.905) centre (-7.2118, -9.1405) ccw
  line L8 (-6.9716, -9.3202) -> (-7.0357, -9.4059)
  spline S8 degree 5 poles (-7.0357, -9.4059) (-7.0387, -9.41) (-7.0448, -9.4183) (-7.0535, -9.4309) (-7.0645, -9.4481) (-7.0775, -9.4701) (-7.0898, -9.4926) (-7.1018, -9.5153) (-7.1136, -9.5381) (-7.1253, -9.5611) (-7.1369, -9.5841) (-7.1482, -9.6073) (-7.1594, -9.6306) (-7.1702, -9.6541) (-7.1808, -9.6778) (-7.191, -9.7017) (-7.2011, -9.7258) (-7.2109, -9.7499) (-7.2206, -9.7742) (-7.2302, -9.7986) (-7.2395, -9.8231) (-7.2487, -9.8476) (-7.2577, -9.8723) (-7.2666, -9.8971) (-7.2752, -9.9221) (-7.2837, -9.9471) (-7.292, -9.9722) (-7.3002, -9.9974) (-7.3081, -10.0227) (-7.316, -10.0481) (-7.3237, -10.0736) (-7.3312, -10.0992) (-7.3386, -10.1249) (-7.3459, -10.1506) (-7.3529, -10.1765) (-7.3599, -10.2024) (-7.3667, -10.2284) (-7.3733, -10.2545) (-7.3799, -10.2806) (-7.3862, -10.3068) (-7.3925, -10.3332) (-7.3986, -10.3595) (-7.4045, -10.386) (-7.4104, -10.4125) (-7.416, -10.4391) (-7.4216, -10.4658) (-7.427, -10.4925) (-7.4323, -10.5193) (-7.4375, -10.5462) (-7.4425, -10.5731) (-7.4474, -10.6002) (-7.4522, -10.6272) (-7.4568, -10.6544) (-7.4614, -10.6815) (-7.4657, -10.7088) (-7.47, -10.7361) (-7.4741, -10.7635) (-7.4782, -10.7909) (-7.4821, -10.8184) (-7.4858, -10.846) (-7.4895, -10.8736) (-7.493, -10.9012) (-7.4964, -10.929) (-7.4997, -10.9567) (-7.5028, -10.9846) (-7.5059, -11.0125) (-7.5088, -11.0404) (-7.5116, -11.0684) (-7.5142, -11.0964) (-7.5168, -11.1245) (-7.5192, -11.1526) (-7.5211, -11.1752) (-7.5224, -11.1921) (-7.5233, -11.2034) (-7.5237, -11.2091) knots 0 0 0 0 0 0 0.01428571 0.02857143 0.04285714 0.05714286 0.07142857 0.08571429 0.1 0.11428571 0.12857143 0.14285714 0.15714286 0.17142857 0.18571429 0.2 0.21428571 0.22857143 0.24285714 0.25714286 0.27142857 0.28571429 0.3 0.31428571 0.32857143 0.34285714 0.35714286 0.37142857 0.38571429 0.4 0.41428571 0.42857143 0.44285714 0.45714286 0.47142857 0.48571429 0.5 0.51428571 0.52857143 0.54285714 0.55714286 0.57142857 0.58571429 0.6 0.61428571 0.62857143 0.64285714 0.65714286 0.67142857 0.68571429 0.7 0.71428571 0.72857143 0.74285714 0.75714286 0.77142857 0.78571429 0.8 0.81428571 0.82857143 0.84285714 0.85714286 0.87142857 0.88571429 0.9 0.91428571 0.92857143 0.94285714 0.95714286 0.97142857 0.98571429 1 1 1 1 1 1
  arc A18 (-7.5237, -11.2091) -> (-6.9388, -11.5803) centre (0, 0) ccw
  spline S9 degree 5 poles (-6.9388, -11.5803) (-6.9339, -11.5775) (-6.924, -11.5719) (-6.9093, -11.5635) (-6.8897, -11.5522) (-6.8653, -11.538) (-6.8409, -11.5237) (-6.8167, -11.5094) (-6.7926, -11.4949) (-6.7685, -11.4804) (-6.7446, -11.4658) (-6.7208, -11.451) (-6.697, -11.4363) (-6.6734, -11.4214) (-6.6499, -11.4064) (-6.6264, -11.3914) (-6.6031, -11.3762) (-6.5799, -11.361) (-6.5568, -11.3457) (-6.5338, -11.3303) (-6.5109, -11.3148) (-6.4881, -11.2992) (-6.4654, -11.2835) (-6.4428, -11.2678) (-6.4203, -11.2519) (-6.398, -11.236) (-6.3758, -11.22) (-6.3537, -11.2039) (-6.3316, -11.1877) (-6.3098, -11.1714) (-6.288, -11.155) (-6.2664, -11.1385) (-6.2448, -11.122) (-6.2234, -11.1053) (-6.2022, -11.0885) (-6.181, -11.0717) (-6.16, -11.0548) (-6.1391, -11.0377) (-6.1183, -11.0206) (-6.0977, -11.0034) (-6.0772, -10.9861) (-6.0568, -10.9687) (-6.0366, -10.9511) (-6.0165, -10.9335) (-5.9966, -10.9158) (-5.9768, -10.898) (-5.9572, -10.8801) (-5.9377, -10.8621) (-5.9183, -10.844) (-5.8991, -10.8257) (-5.8801, -10.8074) (-5.8612, -10.789) (-5.8426, -10.7704) (-5.8241, -10.7518) (-5.8057, -10.733) (-5.7876, -10.7141) (-5.7696, -10.6951) (-5.7517, -10.676) (-5.7341, -10.6568) (-5.7166, -10.6375) (-5.6994, -10.618) (-5.6824, -10.5983) (-5.6657, -10.5785) (-5.6494, -10.5585) (-5.6332, -10.5384) (-5.6173, -10.5181) (-5.6015, -10.4978) (-5.5859, -10.4773) (-5.5704, -10.4568) (-5.5554, -10.436) (-5.5409, -10.4149) (-5.5301, -10.3976) (-5.5224, -10.3844) (-5.5175, -10.3754) (-5.5151, -10.3709) knots -1 -1 -1 -1 -1 -1 -0.98571429 -0.97142857 -0.95714286 -0.94285714 -0.92857143 -0.91428571 -0.9 -0.88571429 -0.87142857 -0.85714286 -0.84285714 -0.82857143 -0.81428571 -0.8 -0.78571429 -0.77142857 -0.75714286 -0.74285714 -0.72857143 -0.71428571 -0.7 -0.68571429 -0.67142857 -0.65714286 -0.64285714 -0.62857143 -0.61428571 -0.6 -0.58571429 -0.57142857 -0.55714286 -0.54285714 -0.52857143 -0.51428571 -0.5 -0.48571429 -0.47142857 -0.45714286 -0.44285714 -0.42857143 -0.41428571 -0.4 -0.38571429 -0.37142857 -0.35714286 -0.34285714 -0.32857143 -0.31428571 -0.3 -0.28571429 -0.27142857 -0.25714286 -0.24285714 -0.22857143 -0.21428571 -0.2 -0.18571429 -0.17142857 -0.15714286 -0.14285714 -0.12857143 -0.11428571 -0.1 -0.08571429 -0.07142857 -0.05714286 -0.04285714 -0.02857143 -0.01428571 0 0 0 0 0 0
  line L9 (-5.5151, -10.3709) -> (-5.4648, -10.2764)
  arc A19 (-5.066, -10.1489) -> (-5.4648, -10.2764) centre (-5.2, -10.4173) ccw
  arc A20 (-5.066, -10.1489) -> (-4.5907, -10.3725) centre (0, 0) ccw
  arc A21 (-4.4347, -10.7612) -> (-4.5907, -10.3725) centre (-4.7121, -10.6469) ccw
  line L10 (-4.4347, -10.7612) -> (-4.4755, -10.8601)
  spline S10 degree 5 poles (-4.4755, -10.8601) (-4.4774, -10.8648) (-4.4812, -10.8743) (-4.4865, -10.8887) (-4.4929, -10.9081) (-4.5, -10.9327) (-4.5064, -10.9575) (-4.5124, -10.9825) (-4.5181, -11.0076) (-4.5237, -11.0327) (-4.5292, -11.0579) (-4.5344, -11.0832) (-4.5394, -11.1085) (-4.5441, -11.134) (-4.5484, -11.1596) (-4.5524, -11.1853) (-4.5562, -11.2111) (-4.5597, -11.2369) (-4.563, -11.2628) (-4.5662, -11.2888) (-4.5692, -11.3148) (-4.572, -11.3409) (-4.5746, -11.3671) (-4.577, -11.3933) (-4.5791, -11.4196) (-4.5811, -11.446) (-4.5829, -11.4724) (-4.5845, -11.4988) (-4.586, -11.5253) (-4.5873, -11.5519) (-4.5884, -11.5785) (-4.5893, -11.6051) (-4.5901, -11.6318) (-4.5907, -11.6586) (-4.5912, -11.6853) (-4.5914, -11.7122) (-4.5916, -11.7391) (-4.5915, -11.766) (-4.5913, -11.7929) (-4.591, -11.8199) (-4.5905, -11.847) (-4.5898, -11.874) (-4.589, -11.9011) (-4.5881, -11.9283) (-4.587, -11.9555) (-4.5857, -11.9827) (-4.5843, -12.0099) (-4.5828, -12.0372) (-4.5811, -12.0645) (-4.5793, -12.0919) (-4.5773, -12.1192) (-4.5752, -12.1466) (-4.5729, -12.1741) (-4.5705, -12.2015) (-4.568, -12.229) (-4.5654, -12.2565) (-4.5626, -12.2841) (-4.5596, -12.3117) (-4.5566, -12.3393) (-4.5534, -12.3669) (-4.55, -12.3945) (-4.5465, -12.4222) (-4.5429, -12.4499) (-4.5392, -12.4776) (-4.5354, -12.5053) (-4.5314, -12.5331) (-4.5272, -12.5609) (-4.523, -12.5887) (-4.5186, -12.6165) (-4.5141, -12.6444) (-4.5095, -12.6722) (-4.5056, -12.6945) (-4.5027, -12.7113) (-4.5008, -12.7224) (-4.4998, -12.728) knots 0 0 0 0 0 0 0.01428571 0.02857143 0.04285714 0.05714286 0.07142857 0.08571429 0.1 0.11428571 0.12857143 0.14285714 0.15714286 0.17142857 0.18571429 0.2 0.21428571 0.22857143 0.24285714 0.25714286 0.27142857 0.28571429 0.3 0.31428571 0.32857143 0.34285714 0.35714286 0.37142857 0.38571429 0.4 0.41428571 0.42857143 0.44285714 0.45714286 0.47142857 0.48571429 0.5 0.51428571 0.52857143 0.54285714 0.55714286 0.57142857 0.58571429 0.6 0.61428571 0.62857143 0.64285714 0.65714286 0.67142857 0.68571429 0.7 0.71428571 0.72857143 0.74285714 0.75714286 0.77142857 0.78571429 0.8 0.81428571 0.82857143 0.84285714 0.85714286 0.87142857 0.88571429 0.9 0.91428571 0.92857143 0.94285714 0.95714286 0.97142857 0.98571429 1 1 1 1 1 1
  arc A22 (-4.4998, -12.728) -> (-3.8409, -12.9421) centre (0, 0) ccw
  spline S11 degree 5 poles (-3.8409, -12.9421) (-3.8369, -12.9381) (-3.8287, -12.9303) (-3.8165, -12.9184) (-3.8003, -12.9026) (-3.7802, -12.8828) (-3.7602, -12.8629) (-3.7403, -12.843) (-3.7205, -12.823) (-3.7008, -12.803) (-3.6813, -12.7828) (-3.6618, -12.7627) (-3.6425, -12.7424) (-3.6233, -12.7222) (-3.6043, -12.7018) (-3.5853, -12.6814) (-3.5665, -12.6609) (-3.5478, -12.6404) (-3.5292, -12.6198) (-3.5108, -12.5992) (-3.4924, -12.5785) (-3.4742, -12.5577) (-3.4562, -12.5369) (-3.4382, -12.5161) (-3.4204, -12.4951) (-3.4027, -12.4741) (-3.3852, -12.4531) (-3.3677, -12.432) (-3.3505, -12.4108) (-3.3333, -12.3896) (-3.3163, -12.3683) (-3.2994, -12.347) (-3.2827, -12.3256) (-3.2661, -12.3041) (-3.2497, -12.2826) (-3.2334, -12.261) (-3.2172, -12.2394) (-3.2012, -12.2177) (-3.1854, -12.1959) (-3.1697, -12.1741) (-3.1541, -12.1523) (-3.1388, -12.1303) (-3.1235, -12.1083) (-3.1085, -12.0863) (-3.0936, -12.0642) (-3.0788, -12.042) (-3.0643, -12.0198) (-3.0499, -11.9975) (-3.0356, -11.9751) (-3.0215, -11.9527) (-3.0077, -11.9302) (-2.994, -11.9077) (-2.9805, -11.885) (-2.9672, -11.8624) (-2.9542, -11.8396) (-2.9413, -11.8168) (-2.9286, -11.7939) (-2.916, -11.771) (-2.9037, -11.748) (-2.8916, -11.7249) (-2.8797, -11.7018) (-2.8682, -11.6785) (-2.857, -11.6552) (-2.8461, -11.6317) (-2.8355, -11.6082) (-2.8251, -11.5846) (-2.8148, -11.561) (-2.8048, -11.5373) (-2.7949, -11.5136) (-2.7855, -11.4897) (-2.7768, -11.4657) (-2.7706, -11.4463) (-2.7664, -11.4315) (-2.7639, -11.4216) (-2.7627, -11.4166) knots -1 -1 -1 -1 -1 -1 -0.98571429 -0.97142857 -0.95714286 -0.94285714 -0.92857143 -0.91428571 -0.9 -0.88571429 -0.87142857 -0.85714286 -0.84285714 -0.82857143 -0.81428571 -0.8 -0.78571429 -0.77142857 -0.75714286 -0.74285714 -0.72857143 -0.71428571 -0.7 -0.68571429 -0.67142857 -0.65714286 -0.64285714 -0.62857143 -0.61428571 -0.6 -0.58571429 -0.57142857 -0.55714286 -0.54285714 -0.52857143 -0.51428571 -0.5 -0.48571429 -0.47142857 -0.45714286 -0.44285714 -0.42857143 -0.41428571 -0.4 -0.38571429 -0.37142857 -0.35714286 -0.34285714 -0.32857143 -0.31428571 -0.3 -0.28571429 -0.27142857 -0.25714286 -0.24285714 -0.22857143 -0.21428571 -0.2 -0.18571429 -0.17142857 -0.15714286 -0.14285714 -0.12857143 -0.11428571 -0.1 -0.08571429 -0.07142857 -0.05714286 -0.04285714 -0.02857143 -0.01428571 0 0 0 0 0 0
  line L11 (-2.7627, -11.4166) -> (-2.7375, -11.3126)
  arc A23 (-2.3829, -11.0899) -> (-2.7375, -11.3126) centre (-2.4459, -11.3832) ccw
  arc A24 (-2.3829, -11.0899) -> (-1.8669, -11.1883) centre (0, 0) ccw
  arc A25 (-1.6192, -11.526) -> (-1.8669, -11.1883) centre (-1.9163, -11.4842) ccw
  line L12 (-1.6192, -11.526) -> (-1.6341, -11.6319)